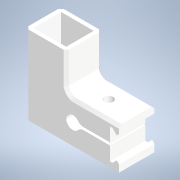
# Autodesk Inventor part: Soporte motor
Saved by Autodesk Inventor 2022 (Build 260153000, 153)
## iProperties
Created: 2021-04-10
Part Number: Soporte motor
Material: ABS Plastic
Document SubType Name: Modeling
Designer: juanp
Density: 1.06 g/cm^3
Appearance: Smooth - White
Author: juanp
Autodesk Inventor part; units mm, degrees
ref_plane "YZ Plane" through (0, 0, 0) normal (1, 0, 0) x (0, 1, 0)
ref_plane "XZ Plane" through (0, 0, 0) normal (0, 1, 0) x (-1, 0, 0)
ref_plane "XY Plane" through (0, 0, 0) normal (0, 0, 1) x (1, 0, 0)
sketch "Sketch1" plane through (0, 0, 0) normal (0, 1, 0) x (-1, 0, 0)
  line L0 (0, 0) -> (12.5, 0)
  line L1 (12.5, 0) -> (12.5, -10.5)
  line L2 (12.5, -10.5) -> (0, -10.5)
  line L3 (0, -10.5) -> (0, 0)
  line L4 (14, 1.5) -> (-1.5, 1.5)
  line L5 (-1.5, 1.5) -> (-1.5, -12)
  line L6 (-1.5, -12) -> (14, -12)
  line L7 (14, -12) -> (14, 1.5)
  line L8 (12.5, 0) -> (0, -10.5) construction
  circle A0 centre (6.25, -5.25) radius 1.75
  dimension "d0" = 12.5
  dimension "d1" = 10.5
  dimension "d2" = 1.5
  dimension "d3" = 1.5
  dimension "d4" = 1.5
  dimension "d5" = 1.5
  dimension "d6" = 3.5
  constraints: 18 end point, 4 parallel, 2 horizontal, 2 perpendicular, 1 centre point, 1 midpoint
  measures "d0" distance of L1.end L2.end
  measures "d1" distance of L0.end L1.end
  measures "d2" distance between parallel lines of L7 L1
  measures "d3" distance between parallel lines of L4 L0
  measures "d4" distance between parallel lines of L3 L5
  measures "d5" distance between parallel lines of L6 L2
  measures "d6" diameter of A0
extrude "Extrusion1" add sketch "Sketch1" along normal blind 1 contours L0 L1 L2 L3
extrude "Extrusion2" add sketch "Sketch1" along normal blind 30 contours L7 L6 L5 L4
sketch "Sketch2" plane through (1.5, 0, -12) normal (0, 0, -1) x (-1, 0, 0)
  line L0 (-2.1986, 29.308) -> (-1.6986, 28.442)
  line L1 (-4.4183, 29.9028) -> (-2.1986, 29.308)
  line L2 (-4.0981, 31.0981) -> (-4.4183, 29.9028)
  line L3 (-12.7583, 26.0981) -> (-4.0981, 31.0981)
  line L4 (-11.5631, 25.7778) -> (-12.7583, 26.0981)
  line L5 (-12.1578, 23.558) -> (-11.5631, 25.7778)
  line L6 (-11.6578, 22.692) -> (-12.1578, 23.558)
  line L7 (-1.6986, 28.442) -> (-11.6578, 22.692)
  line L8 (-12.7583, 26.0981) -> (-15.3564, 24.5981)
  line L9 (-15.3564, 24.5981) -> (-1.1547, 0)
  line L10 (-4.0981, 31.0981) -> (-1.5, 32.5981)
  line L11 (0, 0) -> (0, 30) projected
  line L12 (-6.2452, 25.817) -> (-3.2917, 20.7014)
  line L13 (-4.1578, 20.2014) -> (-7.1112, 25.317)
  line L14 (-7.1112, 25.317) -> (-6.2452, 25.817)
  line L15 (-1.5, 32.5981) -> (0, 30)
  arc A0 (-4.1578, 20.2014) -> (-3.2917, 20.7014) centre (-2.5, 18.3301) ccw
  line L16 (-3.2917, 20.7014) -> (-4.1578, 20.2014) construction
  line L17 (0, 0) -> (0, 30) projected
  line L18 (0, 0) -> (15.5, 0) projected
  line L19 (0, 0) -> (-1.1547, 0)
  point P0 (1.5, 0)
  point P1 (-6.6782, 25.567)
  point P2 (0, 13)
  point P3 (0, 7)
  point P4 (-7.1112, 25.317)
  point P5 (-6.2452, 25.817)
  point P6 (0, 7.5)
  point P7 (0, 18.3301)
  point P8 (-7.1112, 25.317)
  point P9 (-6.2452, 25.817)
  point P10 (0, 18.3301)
  dimension "d12" = 3.5
  dimension "d13" = 11.5
  dimension "d14" = 90
  dimension "d15" = 90
  dimension "d16" = 10
  dimension "d17" = 1
  dimension "d18" = 45
  dimension "d19" = 45
  dimension "d25" = 1
  dimension "d29" = 2.5
  dimension "d42" = 16
  dimension "d46" = 30
  constraints: 34 end point, 4 equal length, 3 parallel, 3 perpendicular, 3 point on line, 2 collinear, 2 midpoint, 2 point on circle, 1 centre point, 1 horizontal, 1 tangent
  measures "d12" distance between parallel lines of L3 L7
  measures "d13" distance between parallel lines of L0 L6
  measures "d14" angle of L5 L4
  measures "d15" angle of L1 L2
  measures "d16" distance of L3.start L2.start
  measures "d17" distance of L0.start L0.end
  measures "d18" angle of L3 L4
  measures "d19" angle of L2 L3
  measures "d25" distance of L12.end L13.start
  measures "d29" radius of A0
  measures "d42" distance between parallel lines of L9 L15
  measures "d46" angle of L11 L9
extrude "Extrusion3" add sketch "Sketch2" against normal up to surface (13.5 mm away) contours L1 L2 L10 L15 L11 A0 L12 L7 L0 | L13 A0 L11 L19 L9 L8 L4 L5 L6 L7
sketch "Sketch3" plane through (2.366, -0.5, -12) normal (0.8660254, -0.5, 0) x (0.5, 0.8660254, 0)
  line L0 (25.4808, 0) -> (19.5738, 13.5) construction
  circle A0 centre (22.5273, 6.75) radius 1.65
  line L1 (-7.75, 13.5) -> (0.5774, 13.5) projected
  line L2 (25.4808, 0) -> (25.4808, 13.5) projected
  line L3 (25.4808, 13.5) -> (19.5738, 13.5) projected
  line L4 (19.5738, 0) -> (19.5738, 13.5) projected
  line L5 (25.4808, 0) -> (19.5738, 0) projected
  line L6 (25.4808, 0) -> (25.4808, 13.5) projected
  dimension "d22" = 3.3
  constraints: 2 end point, 1 centre point, 1 midpoint
  measures "d22" diameter of A0
extrude "Extrusion4" cut sketch "Sketch3" against normal up to surface contours A0 surface through (0, 0, -10.5) normal (-1, 0, 0)
fillet "Fillet2" radius 3 2 edges at (4.7917, 20.7014, -5.25) (5.6578, 20.2014, -5.25)
chamfer "Chamfer1" distance 1 angle 45 4 edges at (-14, 15, -12) (-14, 15, 1.5) (2.25, 31.299, 1.5) (2.25, 31.299, -12)
sketch "Sketch4" plane through (-0.0129, 27.3796, -5.25) normal (-0.8660254, 0.5, 0) x (0, 0, 1)
  line L0 (1.6108, 2.3623) -> (3.2216, -0.4277)
  line L1 (3.2216, -0.4277) -> (1.6108, -3.2177)
  line L2 (1.6108, -3.2177) -> (-1.6108, -3.2177)
  line L3 (-1.6108, -3.2177) -> (-3.2216, -0.4277)
  line L4 (-3.2216, -0.4277) -> (-1.6108, 2.3623)
  line L5 (-1.6108, 2.3623) -> (1.6108, 2.3623)
  circle A0 centre (0, -0.4277) radius 1.65 projected
  point P0 (5.25, -23.705)
  dimension "d37" = 5.58
  constraints: 12 end point, 1 coincident, 1 horizontal, 13 other
  measures "d37" distance between parallel lines of L5 L2
extrude "Extrusion5" cut sketch "Sketch4" against normal blind 4.4 contours L0 L1 L2 L3 L4 L5 | A0
extrude "Extrusion6" cut sketch "Sketch4" along normal blind 10 contours L0 L1 L2 L3 L4 L5 | A0
fillet "Fillet4" radius 1 2 edges at (0, 30, -1.7946) (0, 30, -8.7054)
body "Solid1"
